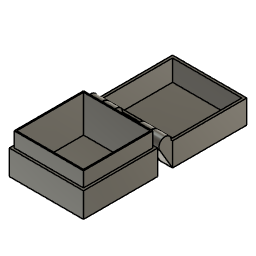
Case test (Autodesk Fusion 360 design; units mm, degrees)
Autodesk Fusion 360 part; units mm, degrees
sketch "Sketch1" plane through (0, 0, 0) normal (0, 0, 1) x (1, 0, 0)
  line L0 (0, 0) -> (30, 0)
  line L1 (30, 0) -> (30, 30)
  line L2 (30, 30) -> (0, 30)
  line L3 (0, 30) -> (0, 0)
  line L4 (1, 29) -> (29, 29)
  line L5 (29, 29) -> (29, 1)
  line L6 (29, 1) -> (1, 1)
  line L7 (1, 1) -> (1, 29)
  constraint horizontal L0
  constraint vertical L1
  constraint horizontal L2
  constraint vertical L3
  constraint coincident L0.start L3.end
  constraint horizontal L4
  constraint vertical L5
  constraint horizontal L6
  constraint vertical L7
extrude "Extrude1" add sketch "Sketch1" along normal blind 1 contours L0 L1 L2 L3 | L4 L5 L6 L7 makes body 1
extrude "Extrude2" add sketch "Sketch1" along normal blind 10 bodies 1
ref_plane "WorkPlane1" through (15, -3, 5) normal (0, -1, 0) x (1, 0, 0)
mirror "Mirror1" about plane through (15, -3, 5) normal (0, -1, 0) of bodies 1 makes body 2
sketch "Sketch2" plane through (30, 0, 0) normal (1, 0, 0) x (0, 1, 0)
  line L0 (0, 0) -> (30, 0)
  line L1 (30, 0) -> (30, 10)
  line L2 (30, 10) -> (0, 10)
  line L3 (0, 10) -> (0, 0)
  line L4 (0, 10) -> (-3, 10)
  circle A0 centre (-3, 10) radius 2.5
  line L5 (0, 0) -> (-5.1529, 8.7291)
  constraint coincident L2.end L3.start
  constraint perpendicular L3 L4
  constraint coincident L4.end A0.centre
  constraint coincident L0.start L3.end
  constraint coincident A0 L5.end
  constraint tangent A0 L5
extrude "Extrude3" add sketch "Sketch2" against normal blind 5 separate body contours L3 L4 A0 L5 | A0 makes body 3
sketch "Sketch3" plane through (25, 0, 0) normal (-1, 0, 0) x (0, -1, 0)
  line L0 (0.5, 10) -> (0, 10)
  line L1 (0, 10) -> (0, 0)
  line L2 (0, 0) -> (5.1529, 8.7291)
  arc A0 (5.1529, 8.7291) -> (0.5, 10) centre (3, 10) ccw
  arc A1 (5.1529, 8.7291) -> (0.5, 10) centre (3, 10) ccw
  circle A2 centre (3, 10) radius 1.5
  constraint concentric A1 A2
extrude "Extrude4" add sketch "Sketch3" along normal blind 3 draft -15 contours A2 bodies 3
fillet "Fillet1" radius 0.75 1 edges at (22, -2.351, 10.2517) on bodies 3
ref_plane "WorkPlane2" through (25, -3.0229, 6.4737) normal (-1, 0, 0) x (0, -1, 0)
sketch "Sketch5" plane through (25, 0, 0) normal (-1, 0, 0) x (0, -1, 0)
  line L0 (6, 10) -> (3, 10)
  circle A0 centre (3, 10) radius 2.5
  line L1 (6, 10) -> (6, 0)
  line L2 (6, 0) -> (0.8471, 8.7291)
  constraint horizontal L0
  constraint coincident L0.end A0.centre
  constraint perpendicular L0 L1
  constraint coincident A0 L2.end
  constraint tangent A0 L2
extrude "Extrude5" add sketch "Sketch5" along normal blind 5.2 and the other way blind -0.2 separate body makes body 4
combine "Combine1" operation cut target body 4 tool bodies 3 keep tools
move_face "OffsetFaces1" offset -0.2 3 faces at (22, -3.0362, 9.9825) (22.4867, -3.7839, 9.7496) (24.426, -4.2129, 10.5841) on bodies 4
ref_plane "WorkPlane3" through (15, -21, 5) normal (1, 0, 0) x (0, -1, 0)
mirror "Mirror2" about plane through (15, -21, 5) normal (1, 0, 0) of bodies 4 3 makes body 5 at (3.3333, -1.7176, 2.9097) makes body 6 at (6.8667, -4.2824, 2.9097)
sketch "Sketch6" plane through (0, 0, 1) normal (0, 0, 1) x (-1, 0, 0)
  line L0 (-29, 35) -> (-29, 7)
  line L1 (-29, 7) -> (-1, 7)
  line L2 (-1, 7) -> (-1, 35)
  line L3 (-1, 35) -> (-29, 35)
  line L4 (-28.5, 7.5) -> (-1.5, 7.5)
  line L5 (-1.5, 7.5) -> (-1.5, 34.5)
  line L6 (-1.5, 34.5) -> (-28.5, 34.5)
  line L7 (-28.5, 34.5) -> (-28.5, 7.5)
  line L8 (-1, 35) -> (-29, 35)
  line L9 (-29, 35) -> (-29, 7)
  line L10 (-29, 7) -> (-1, 7)
  line L11 (-1, 7) -> (-1, 35)
  constraint horizontal L4
  constraint vertical L5
  constraint horizontal L6
  constraint vertical L7
  constraint horizontal L8
  constraint vertical L9
  constraint horizontal L10
  constraint vertical L11
  constraint coincident L0.end L1.start
  constraint coincident L2.end L3.start
extrude "Extrude6" add sketch "Sketch6" along normal blind 15 bodies 2
extrude "Extrude7" cut 1 faces at (0.3333, 19.6667, 10) along direction (0, 0, -1) blind 0.5 on bodies 1 bodies 1
chamfer "Chamfer1" distance 0.5 angle 45 2 edges at (27.5, 0, 10) (2.5, 0, 10) on bodies 3 5
